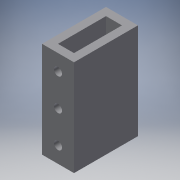
# Autodesk Inventor part: 2AM-17-03-Frame Block
Saved by Autodesk Inventor 2017 (Build 210142000, 142)
## iProperties
Created: 2017-12-29
Part Number: 2AM-17-03-Frame Block
Material: Generic
Document SubType Name: Modeling
Designer: anikasoojin
Density: 1 g/cm^3
Appearance: Default
Author: anikasoojin
Autodesk Inventor part; units mm, degrees
ref_plane "YZ Plane" through (0, 0, 0) normal (1, 0, 0) x (0, 1, 0)
ref_plane "XZ Plane" through (0, 0, 0) normal (0, 1, 0) x (-1, 0, 0)
ref_plane "XY Plane" through (0, 0, 0) normal (0, 0, 1) x (1, 0, 0)
sketch "Sketch1" plane through (0, 0, 0) normal (0, 0, 1) x (1, 0, 0)
  line L0 (-143.1734, 18.1767) -> (-117.7734, 18.1767)
  line L1 (-117.7734, 18.1767) -> (-117.7734, 94.3767)
  line L2 (-117.7734, 94.3767) -> (-143.1734, 94.3767)
  line L3 (-143.1734, 94.3767) -> (-143.1734, 18.1767)
  point P0 (0, 0)
  dimension "d0" = 76.2
  dimension "d1" = 25.4
  constraints: 8 end point, 2 parallel, 1 horizontal, 1 perpendicular
  measures "d0" distance of L2.end L0.start
  measures "d1" distance of L1.end L2.end
extrude "Extrusion1" add sketch "Sketch1" along normal blind 50.8
sketch "Sketch2" plane through (-143.1734, 94.3767, 0) normal (0, 1, 0) x (1, 0, 0)
  line L0 (25.4, 0) -> (0, 0) projected
  line L1 (0, 0) -> (0, -50.8) projected
  line L2 (25.4, -50.8) -> (0, -50.8) projected
  line L3 (25.4, 0) -> (25.4, -50.8) projected
  line L4 (6.35, -44.45) -> (6.35, -6.35)
  line L5 (6.35, -6.35) -> (19.05, -6.35)
  line L6 (19.05, -6.35) -> (19.05, -44.45)
  line L7 (19.05, -44.45) -> (6.35, -44.45)
  point P0 (143.1734, 0)
  dimension "d4" = 6.35
  constraints: 8 end point, 3 other
  measures "d4" distance between parallel lines of L1 L4
extrude "Extrusion2" cut sketch "Sketch2" against normal through all contours L4 L5 L6 L7
sketch "Sketch3" plane through (0, 0, 0) normal (0, 0, -1) x (-1, 0, 0)
  line L0 (143.1734, 18.1767) -> (117.7734, 18.1767) projected
  line L1 (130.4734, 18.1767) -> (130.4734, 94.3767) construction
  line L2 (136.8234, 94.3767) -> (124.1234, 94.3767) projected
  circle A0 centre (130.4734, 30.8767) radius 3.175
  circle A1 centre (130.4734, 56.2767) radius 3.175
  circle A2 centre (130.4734, 81.6767) radius 3.175
  point P0 (0, 0)
  dimension "d7" = 6.35
  dimension "d8" = 12.7
  dimension "d11" = 25.4
  constraints: 3 centre point, 2 end point, 2 midpoint, 1 point on line, 1 vertical, 4 other
  measures "d7" diameter of A0
  measures "d8" distance of L1.start A0.centre
  measures "d11" distance of A0.centre A1.centre
extrude "Extrusion3" cut sketch "Sketch3" against normal through all
body "Solid1"
